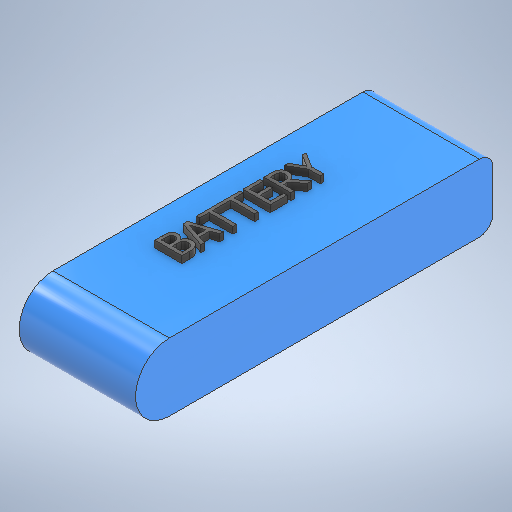
# Autodesk Inventor part: 3S Lipo Battery - 11.1 V
Saved by Autodesk Inventor 2025.2 (Build 292293000, 293)
## iProperties
Created: 2025-01-24
Part Number: 3S Lipo Battery - 11.1 V
Material: Generic
Document SubType Name: Modeling
Designer: Matt Tidd
Density: 1 g/cm^3
Appearance: Default
Author: Matt Tidd
Autodesk Inventor part; units mm, degrees
ref_plane "YZ Plane" through (0, 0, 0) normal (1, 0, 0) x (0, 1, 0)
ref_plane "XZ Plane" through (0, 0, 0) normal (0, 1, 0) x (-1, 0, 0)
ref_plane "XY Plane" through (0, 0, 0) normal (0, 0, 1) x (1, 0, 0)
sketch "Sketch1" plane through (0, 0, 0) normal (0, 1, 0) x (-1, 0, 0)
  line L0 (0, 0) -> (43, 0)
  line L1 (43, 0) -> (43, -132)
  line L2 (43, -132) -> (0, -132)
  line L3 (0, -132) -> (0, 0)
  dimension "d0" = 43
  dimension "d1" = 132
  constraints: 8 end point, 2 parallel, 1 horizontal, 1 perpendicular
  measures "d0" distance of L1.end L2.end
  measures "d1" distance of L0.end L1.end
extrude "Extrusion1" add sketch "Sketch1" along normal blind 25
fillet "Fillet1" radius 12.5 2 edges at (-21.5, 25, 0) (-21.5, 0, 0)
fillet "Fillet2" radius 5 2 edges at (-21.5, 25, -132) (-21.5, 0, -132)
sketch "Sketch2" plane through (0, 25, 0) normal (0, 1, 0) x (1, 0, 0)
  line L0 (0, 132) -> (-43, 132) construction
  line L1 (-21.5, 132) -> (-21.5, 0) construction
  line L2 (0, 12.5) -> (0, 127) construction
  line L3 (0, 66) -> (-43, 66) construction
  spline S0 degree 2 poles (-24.5713, 45.4206) (-23.8258, 45.4206) (-22.6831, 44.8533) (-22.3104, 44.3833) knots 0 0 0 1 2 2 2
  spline S1 degree 2 poles (-22.3104, 44.3833) (-21.8728, 43.816) (-21.5, 42.5276) (-21.5, 41.5065) knots 0 0 0 1 2 2 2
  line L4 (-21.5, 41.5065) -> (-21.5, 38.6378)
  line L5 (-21.5, 38.6378) -> (-31.5, 38.6378)
  line L6 (-31.5, 38.6378) -> (-31.5, 41.2877)
  spline S2 degree 2 poles (-31.5, 41.2877) (-31.5, 42.3574) (-31.3622, 43.4271) (-31.0948, 43.9133) knots 0 0 0 1 2 2 2
  spline S3 degree 2 poles (-31.0948, 43.9133) (-30.8112, 44.4562) (-29.8793, 44.9506) (-29.2472, 44.9506) knots 0 0 0 1 2 2 2
  spline S4 degree 2 poles (-29.2472, 44.9506) (-28.5421, 44.9506) (-27.4238, 44.205) (-27.1078, 43.5486) knots 0 0 0 1 2 2 2
  line L7 (-27.1078, 43.5486) -> (-27.0592, 43.5486)
  spline S5 degree 2 poles (-27.0592, 43.5486) (-26.816, 44.44) (-25.5276, 45.4206) (-24.5713, 45.4206) knots 0 0 0 1 2 2 2
  spline S6 degree 2 poles (-24.5146, 44.0348) (-25.0818, 44.0348) (-25.8112, 43.7107) (-26.0705, 43.2245) knots 0 0 0 1 2 2 2
  spline S7 degree 2 poles (-26.0705, 43.2245) (-26.2326, 42.9084) (-26.3298, 42.1629) (-26.3298, 41.4741) knots 0 0 0 1 2 2 2
  line L8 (-26.3298, 41.4741) -> (-26.3298, 39.9668)
  line L9 (-26.3298, 39.9668) -> (-22.6345, 39.9668)
  line L10 (-22.6345, 39.9668) -> (-22.6345, 41.0446)
  spline S8 degree 2 poles (-22.6345, 41.0446) (-22.6345, 41.9198) (-22.7966, 42.9246) (-23.0559, 43.3136) knots 0 0 0 1 2 2 2
  spline S9 degree 2 poles (-23.0559, 43.3136) (-23.3233, 43.6864) (-23.9878, 44.0348) (-24.5146, 44.0348) knots 0 0 0 1 2 2 2
  spline S10 degree 2 poles (-29.0608, 43.5648) (-29.4173, 43.5648) (-29.9522, 43.3217) (-30.1062, 43.0543) knots 0 0 0 1 2 2 2
  spline S11 degree 2 poles (-30.1062, 43.0543) (-30.2844, 42.7301) (-30.3655, 41.9441) (-30.3655, 41.2391) knots 0 0 0 1 2 2 2
  line L11 (-30.3655, 41.2391) -> (-30.3655, 39.9668)
  line L12 (-30.3655, 39.9668) -> (-27.44, 39.9668)
  line L13 (-27.44, 39.9668) -> (-27.44, 41.4741)
  spline S12 degree 2 poles (-27.44, 41.4741) (-27.44, 42.0981) (-27.5697, 42.6896) (-27.7723, 43.0057) knots 0 0 0 1 2 2 2
  spline S13 degree 2 poles (-27.7723, 43.0057) (-27.9668, 43.3136) (-28.5908, 43.5648) (-29.0608, 43.5648) knots 0 0 0 1 2 2 2
  line L14 (-21.5, 45.6637) -> (-31.5, 49.0348)
  line L15 (-31.5, 49.0348) -> (-31.5, 50.6718)
  line L16 (-31.5, 50.6718) -> (-21.5, 54.043)
  line L17 (-21.5, 54.043) -> (-21.5, 52.641)
  line L18 (-21.5, 52.641) -> (-24.2958, 51.7334)
  line L19 (-24.2958, 51.7334) -> (-24.2958, 47.9165)
  line L20 (-24.2958, 47.9165) -> (-21.5, 47.0089)
  line L21 (-21.5, 47.0089) -> (-21.5, 45.6637)
  line L22 (-25.4303, 51.3687) -> (-30.1386, 49.8209)
  line L23 (-30.1386, 49.8209) -> (-25.4303, 48.2812)
  line L24 (-25.4303, 48.2812) -> (-25.4303, 51.3687)
  line L25 (-21.5, 57.4546) -> (-30.3169, 57.4546)
  line L26 (-30.3169, 57.4546) -> (-30.3169, 54.0997)
  line L27 (-30.3169, 54.0997) -> (-31.5, 54.0997)
  line L28 (-31.5, 54.0997) -> (-31.5, 62.1386)
  line L29 (-31.5, 62.1386) -> (-30.3169, 62.1386)
  line L30 (-30.3169, 62.1386) -> (-30.3169, 58.7836)
  line L31 (-30.3169, 58.7836) -> (-21.5, 58.7836)
  line L32 (-21.5, 58.7836) -> (-21.5, 57.4546)
  line L33 (-21.5, 65.4935) -> (-30.3169, 65.4935)
  line L34 (-30.3169, 65.4935) -> (-30.3169, 62.1386)
  line L35 (-30.3169, 62.1386) -> (-31.5, 62.1386)
  line L36 (-31.5, 62.1386) -> (-31.5, 70.1775)
  line L37 (-31.5, 70.1775) -> (-30.3169, 70.1775)
  line L38 (-30.3169, 70.1775) -> (-30.3169, 66.8225)
  line L39 (-30.3169, 66.8225) -> (-21.5, 66.8225)
  line L40 (-21.5, 66.8225) -> (-21.5, 65.4935)
  line L41 (-21.5, 71.1985) -> (-31.5, 71.1985)
  line L42 (-31.5, 71.1985) -> (-31.5, 77.4546)
  line L43 (-31.5, 77.4546) -> (-30.3169, 77.4546)
  line L44 (-30.3169, 77.4546) -> (-30.3169, 72.5276)
  line L45 (-30.3169, 72.5276) -> (-27.5778, 72.5276)
  line L46 (-27.5778, 72.5276) -> (-27.5778, 77.1224)
  line L47 (-27.5778, 77.1224) -> (-26.3947, 77.1224)
  line L48 (-26.3947, 77.1224) -> (-26.3947, 72.5276)
  line L49 (-26.3947, 72.5276) -> (-22.6831, 72.5276)
  line L50 (-22.6831, 72.5276) -> (-22.6831, 77.4546)
  line L51 (-22.6831, 77.4546) -> (-21.5, 77.4546)
  line L52 (-21.5, 77.4546) -> (-21.5, 71.1985)
  line L53 (-21.5, 86.6524) -> (-21.5, 84.9263)
  line L54 (-21.5, 84.9263) -> (-25.4789, 81.7658)
  line L55 (-25.4789, 81.7658) -> (-25.4789, 80.2423)
  line L56 (-25.4789, 80.2423) -> (-21.5, 80.2423)
  line L57 (-21.5, 80.2423) -> (-21.5, 78.9133)
  line L58 (-21.5, 78.9133) -> (-31.5, 78.9133)
  line L59 (-31.5, 78.9133) -> (-31.5, 81.4903)
  spline S14 degree 2 poles (-31.5, 81.4903) (-31.5, 82.3493) (-31.3136, 83.5081) (-30.9733, 84.0348) knots 0 0 0 1 2 2 2
  spline S15 degree 2 poles (-30.9733, 84.0348) (-30.6329, 84.5616) (-29.5713, 85.1694) (-28.7853, 85.1694) knots 0 0 0 1 2 2 2
  spline S16 degree 2 poles (-28.7853, 85.1694) (-27.6912, 85.1694) (-26.2083, 84.0511) (-25.8517, 83.0948) knots 0 0 0 1 2 2 2
  line L60 (-25.8517, 83.0948) -> (-21.5, 86.6524)
  spline S17 degree 2 poles (-28.6799, 83.7836) (-29.1175, 83.7836) (-29.7901, 83.4757) (-30.0089, 83.1515) knots 0 0 0 1 2 2 2
  spline S18 degree 2 poles (-30.0089, 83.1515) (-30.1953, 82.8679) (-30.3493, 82.1143) (-30.3493, 81.5632) knots 0 0 0 1 2 2 2
  line L61 (-30.3493, 81.5632) -> (-30.3493, 80.2423)
  line L62 (-30.3493, 80.2423) -> (-26.5891, 80.2423)
  line L63 (-26.5891, 80.2423) -> (-26.5891, 81.4092)
  spline S19 degree 2 poles (-26.5891, 81.4092) (-26.5891, 81.9846) (-26.7917, 82.9003) (-27.1078, 83.2164) knots 0 0 0 1 2 2 2
  spline S20 degree 2 poles (-27.1078, 83.2164) (-27.3833, 83.5081) (-28.1613, 83.7836) (-28.6799, 83.7836) knots 0 0 0 1 2 2 2
  line L64 (-31.5, 94.4481) -> (-25.9246, 91.0689)
  line L65 (-25.9246, 91.0689) -> (-21.5, 91.0689)
  line L66 (-21.5, 91.0689) -> (-21.5, 89.7399)
  line L67 (-21.5, 89.7399) -> (-25.7869, 89.7399)
  line L68 (-25.7869, 89.7399) -> (-31.5, 86.3606)
  line L69 (-31.5, 86.3606) -> (-31.5, 87.8355)
  line L70 (-31.5, 87.8355) -> (-27.0997, 90.4125)
  line L71 (-27.0997, 90.4125) -> (-31.5, 93.0381)
  line L72 (-31.5, 93.0381) -> (-31.5, 94.4481)
  point P0 (0, 0)
  constraints: 4 end point, 2 vertical, 1 horizontal, 1 midpoint, 1 point on line
extrude "Extrusion2" add sketch "Sketch2" along normal blind 2.5
body "Solid1"
